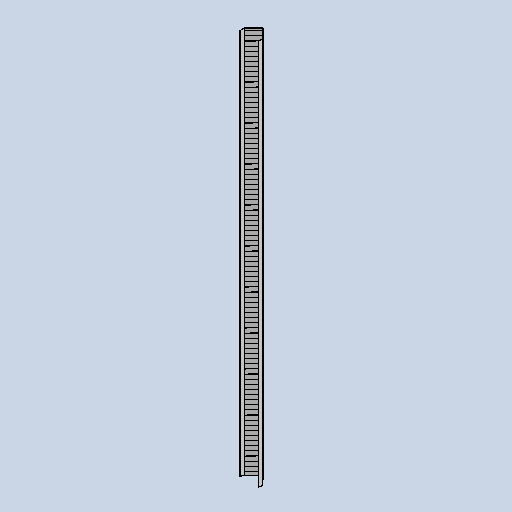
# Autodesk Inventor part: DSB-512 roof 2
Saved by Autodesk Inventor 2025.1 (Build 291241020, 241B)
## iProperties
Created: 2024-07-24
Part Number: DSB-512 roof 2
Material: Stainless Steel
Document SubType Name: Sheet Metal
Designer: admin
Density: 8 g/cm^3
Flat Pattern Width: 7.85084 cm
Flat Pattern Length: 87.5 cm
Flat Pattern Area: 686.948 cm^2
Sheet Metal Rule: Default
Sheet Metal Width: 78.508 mm
Sheet Metal Length: 875.000 mm
Sheet Metal Area: 68694.822 mm^2
Appearance: Default
Author: admin
Autodesk Inventor part; units mm, degrees
note: some values were not read from the file. Chosen so that the rebuilt part matches the saved one: flange form of "Plate1".
ref_plane "YZ Plane" through (0, 0, 0) normal (1, 0, 0) x (0, 1, 0)
ref_plane "XZ Plane" through (0, 0, 0) normal (0, 1, 0) x (-1, 0, 0)
ref_plane "XY Plane" through (0, 0, 0) normal (0, 0, 1) x (1, 0, 0)
sketch "Sketch3" plane through (0, 0, 0) normal (0, 0, 1) x (1, 0, 0)
  line L0 (-21, -10) -> (-21, -0.404026)
  line L1 (-21, 0) -> (-20.71934, 0.290632) construction
  line L2 (0, 21.746137) -> (0.71934, 21.001238) construction
  line L3 (21, 0) -> (21, -0.404026) construction
  line L4 (0, 21.746137) -> (0, 0) construction
  arc A0 (0.71934, 21.001238) -> (-0.71934, 21.001238) centre (0, 20.30658) ccw
  arc A1 (-20.71934, 0.290632) -> (-21, -0.404026) centre (-20, -0.404026) ccw
  arc A2 (21, -0.404026) -> (20.71934, 0.290632) centre (20, -0.404026) ccw
  line L5 (20.71934, 0.290632) -> (21, 0) construction
  line L6 (21, -0.404026) -> (21, -10)
  line L7 (-20.71934, 0.290632) -> (-0.71934, 21.001238)
  line L8 (-21, -0.404026) -> (-21, 0) construction
  line L9 (0.71934, 21.001238) -> (20.71934, 0.290632)
  line L10 (-0.71934, 21.001238) -> (0, 21.746137) construction
  dimension "d15" = 10
  dimension "d18" = 1
  dimension "d19" = 1
  dimension "d20" = 1
  dimension "d32" = 42
  dimension "d33" = 88
  measures "d15" distance of L3.start L6.end
  measures "d18" radius of A0
  measures "d19" radius of A1
  measures "d20" radius of A2
  measures "d32" distance between parallel lines of L6 L0
  measures "d33" angle of L9 L7
contour flange "Contour Flange1" sketch "Sketch3" thickness 0.8 bend radius 0.8 width 875 along (0, 0, -1) mid plane no both sides no wall seen from (-21, -5.202013, 0) lies toward (1, 0, 0) curves L0 A1 L7 A0 L9 A2 L6
bend "Bend1"
corner "Corner1"
sketch "Sketch5" plane through (20.71934, 0.290632, 0) normal (0.7193398, 0.6946584, 0) x (-0.6946584, 0.7193398, 0)
  line L0 (0, -875) -> (0, 0) construction
  line L1 (0, 0) -> (28.791131, 0) construction
  line L2 (28.791131, 0) -> (28.791131, -875) construction
  line L3 (28.791131, -875) -> (0, -875) construction
  line L4 (28.291131, -5.1) -> (0.291131, -5.1) construction
  line L5 (28.291131, -5) -> (0.291131, -5)
  line L6 (0.291131, -5.2) -> (28.291131, -5.2)
  arc A0 (28.291131, -5.2) -> (28.291131, -5) centre (28.291131, -5.1) ccw
  arc A1 (0.291131, -5) -> (0.291131, -5.2) centre (0.291131, -5.1) ccw
  point P0 (14.1838, 0)
  point P1 (14.291131, -5.1)
  dimension "d111" = 0.2
  dimension "d112" = 28
  dimension "d114" = 0.5
  dimension "d97" = 5
  constraints: 10 end point, 4 point on circle, 4 tangent, 2 centre point, 2 parallel, 1 midpoint, 1 perpendicular
  measures "d111" diameter of A1
  measures "d112" distance of L4.start L4.end
  measures "d114" distance from line of L4.start L2
  measures "d97" distance between parallel lines of L5 L1
extrude "Cut3" cut sketch "Sketch5" against normal blind 0.8
sketch "Sketch9" plane through (0, 0, 0) normal (1, 0, 0) x (0, 1, 0)
  line L0 (-0.404026, -875) -> (-0.265095, -875)
  line L1 (21.001238, -875) -> (0.290632, -875)
  line L2 (-0.265095, -875) -> (0.290632, -875)
  line L3 (-0.404026, -875) -> (0.290632, -875)
  line L4 (-0.404026, -875) -> (-10, -875)
  line L5 (-0.404026, -875) -> (-10, -875)
  line L6 (-0.404026, -875) -> (0.290632, -875)
  line L7 (-10, -875) -> (-0.404026, -875)
  line L8 (-10, -875) -> (-0.404026, -875)
  line L9 (-0.404026, -875) -> (-0.265095, -875)
  line L10 (-0.265095, -875) -> (0.290632, -875)
  line L11 (21.001238, -875) -> (21.30658, -875)
  line L12 (-0.265095, -875) -> (20.445512, -875)
  line L13 (20.445512, -875) -> (21.001238, -875)
  line L14 (0.290632, -875) -> (21.001238, -875)
  line L15 (20.445512, -875) -> (20.50658, -875)
  line L16 (20.445512, -875) -> (-0.265095, -875)
  line L17 (20.445512, -875) -> (21.001238, -875)
  line L18 (-0.265095, -875) -> (0.290632, -875)
  line L19 (-0.404026, -875) -> (-0.265095, -875)
  line L20 (-0.404026, -875) -> (0.290632, -875)
  line L21 (20.445512, -875) -> (21.001238, -875)
  line L22 (20.445512, -875) -> (20.445512, -875)
  line L23 (20.445512, -875) -> (21.001238, -875)
  line L24 (21.001238, -875) -> (21.001238, -875)
  line L25 (-0.265095, -875) -> (0.290632, -875)
  line L26 (20.445512, -875) -> (-0.265095, -875)
  line L27 (20.445512, -875) -> (21.001238, -875)
  line L28 (21.001238, -875) -> (0.290632, -875)
  line L29 (20.445512, -875) -> (21.001238, -875)
  line L30 (-0.265095, -875) -> (20.445512, -875)
  line L31 (-0.265095, -875) -> (0.290632, -875)
  line L32 (0.290632, -875) -> (21.001238, -875)
  line L33 (-10, -875) -> (-0.404026, -875)
  line L34 (-10, -875) -> (-0.404026, -875)
  line L35 (-0.265095, -875) -> (-0.404026, -875)
  line L36 (-0.265095, -875) -> (0.290632, -875)
  line L37 (0.290632, -875) -> (-0.404026, -875)
  line L38 (-0.404026, -875) -> (-10, -875)
  line L39 (-0.404026, -875) -> (-10, -875)
  line L40 (-10, 0) -> (-10, -875)
  line L41 (-10, -870.71258) -> (20.50658, -875)
  point P0 (0, 0)
extrude "Extrusion4" cut sketch "Sketch9" along normal through all both and the other way through all
pattern_linear "Rectangular Pattern3" count 87 spacing 10 along (0, 0, -1) of "Cut3"
mirror "Mirror3" about plane through (0, 0, 0) normal (1, 0, 0) of "Cut3", "Rectangular Pattern3"
equation "\"d21\" = Thickness"
equation "\"d22\" = BendReliefWidth"
equation "\"d23\" = BendReliefDepth"
equation "\"d24\" = MinimumRemnant"
equation "\"d25\" = TransitionRadius"
equation "\"d27\" = BendRadius"
equation "\"d29\" = CornerReliefSize"
equation "\"d30\" = GapSize"
equation "\"d31\" = JacobiRadiusSize"
equation "\"BendRadius\" = Thickness"
equation "\"BendReliefWidth\" = Thickness"
equation "\"BendReliefDepth\" = 0.5 * Thickness"
equation "\"CornerReliefSize\" = 4 * Thickness"
equation "\"MinimumRemnant\" = 2 * Thickness"
equation "\"TransitionRadius\" = BendRadius"
equation "\"JacobiRadiusSize\" = BendRadius"
equation "\"GapSize\" = Thickness"
equation "\"grat_thick\" = 0.2"
equation "\"grat_lenth\" = 28"
equation "\"grat_indet_X\" = 5"
equation "\"grat_indet_Y\" = 0.5"
equation "\"Thickness\" = 0.8"
body "Solid2"
